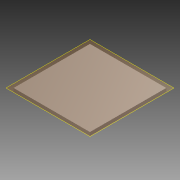
# Autodesk Inventor part: Boden
Saved by Autodesk Inventor 2018.2 (Build 222227000, 227)
## iProperties
Created: 2019-09-20
Part Number: Boden
Material: Generisch
Document SubType Name: Modeling
Designer: Lolob
Density: 1 g/cm^3
Appearance: Vorgabe
Author: Lolob
Autodesk Inventor part; units mm, degrees
ref_plane "YZ Plane" through (0, 0, 0) normal (1, 0, 0) x (0, 1, 0)
ref_plane "XZ Plane" through (0, 0, 0) normal (0, 1, 0) x (-1, 0, 0)
ref_plane "XY Plane" through (0, 0, 0) normal (0, 0, 1) x (1, 0, 0)
ref_plane "Arbeitsebene1" through (-858.9244, 0, 0) normal (0, 0, 1) x (1, 0, 0)
sketch "Skizze2" plane through (-858.9244, 0, 0) normal (0, 0, 1) x (1, 0, 0)
  line L0 (-0.0619, 347.3197) -> (439.9381, 347.3197)
  line L1 (439.9381, 347.3197) -> (439.9381, -92.6803)
  line L2 (439.9381, -92.6803) -> (-0.0619, -92.6803)
  line L3 (-0.0619, -92.6803) -> (-0.0619, 347.3197)
  point P0 (858.9244, 0)
  dimension "d5" = 440
  dimension "d6" = 440
  constraints: 8 end point, 2 parallel, 1 horizontal, 1 perpendicular
  measures "d5" distance of L0.start L0.end
  measures "d6" distance of L0.end L1.end
extrude "Extrusion2" add sketch "Skizze2" along normal blind 20
chamfer "Fase2" distance 20 angle 45 4 edges at (-638.9863, -92.6803, 0) (-418.9863, 127.3197, 0) (-858.9863, 127.3197, 0) (-638.9863, 347.3197, 0)
